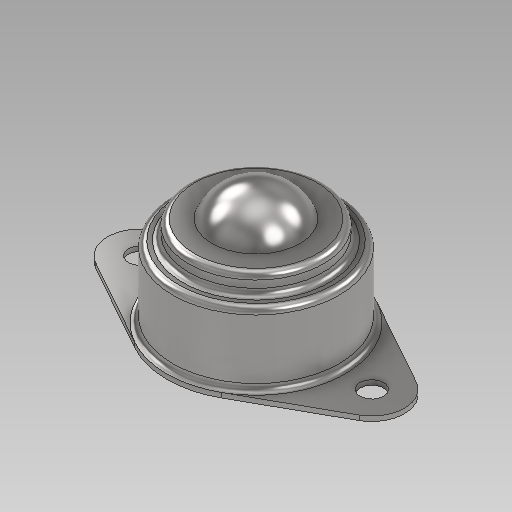
# Autodesk Inventor part: bull_eye_wheel
Saved by Autodesk Inventor 2020 (Build 240168000, 168)
## iProperties
Created: 2020-11-30
Part Number: bull_eye_wheel
Material: Stainless Steel
Document SubType Name: Modeling
Designer: 楊宜瑄
Density: 8 g/cm^3
Appearance: Semi-Polished
Author: 楊宜瑄
Autodesk Inventor part; units mm, degrees
ref_plane "YZ Plane" through (0, 0, 0) normal (1, 0, 0) x (0, 1, 0)
ref_plane "XZ Plane" through (0, 0, 0) normal (0, 1, 0) x (-1, 0, 0)
ref_plane "XY Plane" through (0, 0, 0) normal (0, 0, 1) x (1, 0, 0)
sketch "Sketch1" plane through (0, 0, 0) normal (0, 0, 1) x (1, 0, 0)
  line L0 (-14, 0) -> (-25, 0)
  line L1 (-25, 0) -> (-25, 0.8)
  line L2 (-25, 0.8) -> (-15, 0.8)
  line L3 (-14, 1.8) -> (-14, 11.7862)
  line L4 (-13, 12.7862) -> (-12.3293, 12.7862)
  line L5 (-11.3293, 13.7862) -> (-11.3293, 15)
  line L6 (-10.3293, 16) -> (0, 16)
  line L7 (0, 16) -> (0, 0)
  circle A0 centre (0, 13.0625) radius 7.9375
  circle A1 centre (0, 13.0625) radius 13.0625 construction
  arc A2 (-15, 0.8) -> (-14, 1.8) centre (-15, 1.8) ccw
  arc A3 (-13, 12.7862) -> (-14, 11.7862) centre (-13, 11.7862) ccw
  arc A4 (-12.3293, 12.7862) -> (-11.3293, 13.7862) centre (-12.3293, 13.7862) ccw
  arc A5 (-10.3293, 16) -> (-11.3293, 15) centre (-10.3293, 15) ccw
  arc A6 (-12.0392, 7.9942) -> (0, 0) centre (0, 13.0625) ccw
  arc A7 (-11.6625, 13.041) -> (0, 1.4) centre (0, 13.0625) ccw
  line L8 (-13, 7.8002) -> (-13, 1)
  arc A8 (-14, 0) -> (-13, 1) centre (-14, 1) ccw
  arc A9 (-12.0392, 7.9942) -> (-13, 7.8002) centre (-12.5, 7.8002) ccw
  dimension "d0" = 14
  dimension "d1" = 15.875
  dimension "d2" = 25
  dimension "d3" = 0.8
  dimension "d4" = 16
  dimension "d5" = 13.0625
  dimension "d6" = 1
  dimension "d8" = 1.4
  dimension "d9" = 1
  dimension "d10" = 0.5
  constraints: 20 point on circle, 19 end point, 13 tangent, 10 centre point, 8 perpendicular, 5 point on line, 3 equal radius, 2 coincident, 2 horizontal, 1 concentric, 1 vertical, 4 other
  measures "d0" distance between parallel lines of L3 L7
  measures "d1" diameter of A0
  measures "d2" distance of L7.end L0.end
  measures "d3" distance of L0.end L1.end
  measures "d4" distance between parallel lines of L0 L6
  measures "d5" distance from line of L0 A0.centre
  measures "d6" radius of A2
  measures "d8" radial gap between concentric circles of A1 A7
  measures "d9" radius of A8
  measures "d10" radius of A9
revolve "Revolution1" add sketch "Sketch1" angle 360 about axis through (0, 16, 0) along (0, -1, 0) picked at (-0.6385, 8.8282) contours L0 L1 L2 A2 L3 A3 L4 A4 A7 L7 A6 A9 L8 A8 | A7 A4 L5 A5 L6 A0 L7 | A0 L6 L7
sketch "Sketch2" plane through (0, 0.8, 0) normal (0, 1, 0) x (1, 0, 0)
  circle A0 centre (19.5, 0) radius 2
  circle A1 centre (-19.5, 0) radius 2
  point P0 (0, 0)
  dimension "d12" = 39
  dimension "d13" = 4
  dimension "d14" = 4
  dimension "d15" = 19.5
  constraints: 2 centre point, 2 horizontal alignment
  measures "d12" distance of A1.centre A0.centre
  measures "d13" diameter of A0
  measures "d14" diameter of A1
  measures "d15" distance of point (0, 0) A0.centre
extrude "Extrusion1" cut sketch "Sketch2" against normal blind 10
sketch "Sketch3" plane through (0, 0.8, 0) normal (0, 1, 0) x (1, 0, 0)
  circle A0 centre (-19.5, 0) radius 5.5
  circle A1 centre (-19.5, 0) radius 2 projected
  circle A2 centre (19.5, 0) radius 5.5
  circle A3 centre (19.5, 0) radius 2 projected
  line L0 (-22.1795, -4.8032) -> (-7.3077, -13.0995)
  line L1 (7.3077, -13.0995) -> (22.1795, -4.8032)
  line L2 (7.3077, 13.0995) -> (22.1795, 4.8032)
  circle A4 centre (0, 0) radius 25 projected
  circle A5 centre (0, 0) radius 15 projected
  line L3 (-22.1795, 4.8032) -> (-7.3077, 13.0995)
  circle A6 centre (0, 0) radius 25
  arc A7 (7.3077, 13.0995) -> (-7.3077, 13.0995) centre (0, 0) ccw
  arc A8 (-7.3077, -13.0995) -> (7.3077, -13.0995) centre (0, 0) ccw
  point P0 (0, -17.1762)
  point P1 (0, 17.1762)
  point P2 (25, 0)
  point P3 (-25, 0)
  constraints: 12 point on circle, 9 tangent, 8 end point, 5 centre point, 4 concentric, 1 coincident, 1 vertical alignment
extrude "Extrusion2" cut sketch "Sketch3" against normal through all contours A0 A4 A2 L2 A5 L3 | L0 A5 L1 A2 A4 A0
sketch "Sketch5" plane through (0, 0, 0) normal (0, 0, 1) x (1, 0, 0)
  circle A0 centre (0, 13.063) radius 7.9375
  line L0 (-7.3077, 0) -> (7.3077, 0) projected
  line L1 (0, 34.7827) -> (0, -0.8114)
  line L2 (10.3293, 16) -> (-10.3293, 16) projected
  line L3 (-7.3741, 16) -> (7.3741, 16)
  line L4 (11.3293, 15) -> (-11.3293, 15) projected
  point P0 (0, 0)
  point P1 (-11.3293, 15)
  point P2 (0, 16)
  point P3 (7.3741, 16)
  point P4 (0, 21.0005)
  dimension "d20" = 13.063
  dimension "d21" = 15.875
  constraints: 4 end point, 2 point on circle, 1 centre point, 1 horizontal, 1 perpendicular, 1 point on line, 1 vertical alignment, 1 other
  measures "d20" distance from line of L0 A0.centre
  measures "d21" diameter of A0
revolve "Revolution2" add sketch "Sketch5" angle 360 about axis through (0, 34.7827, 0) along (0, -1, 0) picked at (4.6154, 16.5527) contours L2 L1 A0
body "Solid1"
